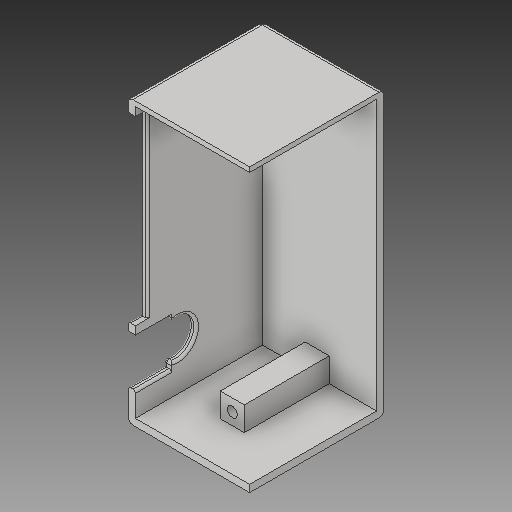
# Autodesk Inventor part: PowerS_cap
Saved by Autodesk Inventor 2019.3 (Build 233278000, 278)
## iProperties
Created: 2020-08-31
Part Number: PowerS_cap
Material: Generisch
Document SubType Name: Modeling
Designer: Nicolas Frick
Density: 1 g/cm^3
Appearance: Vorgabe
Author: Nicolas Frick
Autodesk Inventor part; units mm, degrees
ref_plane "YZ Plane" through (0, 0, 0) normal (1, 0, 0) x (0, 1, 0)
ref_plane "XZ Plane" through (0, 0, 0) normal (0, 1, 0) x (-1, 0, 0)
sketch "Skizze1" plane through (0, 0, 0) normal (0, 0, 1) x (1, 0, 0)
  line L0 (105.8135, 54.6424) -> (-70.1865, 54.6424) construction
  line L1 (-70.1865, 54.6424) -> (-70.1865, -55.3576) construction
  line L2 (-70.1865, -55.3576) -> (-86.1865, -55.3576) construction
  line L3 (-86.1865, -55.3576) -> (-86.1865, -56.6576) construction
  line L4 (112.8344, -56.6576) -> (-86.1865, -56.6576) construction
  line L5 (112.8344, -55.3576) -> (112.8344, -56.6576) construction
  line L6 (112.8344, -55.3576) -> (105.8135, -55.3576) construction
  line L7 (105.8135, -55.3576) -> (105.8135, 54.6424) construction
  line L8 (-104.5712, -45.4245) -> (-104.5712, -55.4245) construction
  line L9 (112.8135, -55.4245) -> (-104.5712, -55.4245) construction
  line L10 (112.8135, 46.962) -> (112.8135, -55.4245) construction
  line L11 (110.3928, 46.962) -> (112.8135, 46.962) construction
  arc A0 (110.3928, 50.262) -> (110.3928, 46.962) centre (110.3928, 48.612) ccw construction
  line L12 (112.8135, 50.262) -> (110.3928, 50.262) construction
  line L13 (112.8135, 54.6424) -> (112.8135, 50.262) construction
  line L14 (-86.7728, 54.6424) -> (112.8135, 54.6424) construction
  line L15 (-86.7728, 54.6424) -> (-86.7728, 44.6424) construction
  line L16 (-86.7728, 44.6424) -> (-96.7728, 44.6424) construction
  line L17 (-96.7728, 44.6424) -> (-96.7728, 54.6424) construction
  line L18 (-112.5712, 54.6424) -> (-96.7728, 54.6424) construction
  arc A1 (-112.5712, 54.6424) -> (-114.5712, 52.6424) centre (-112.5712, 52.6424) ccw construction
  line L19 (-114.5712, 44.6424) -> (-114.5712, 52.6424) construction
  line L20 (-114.5712, 44.6424) -> (-104.5712, 44.6424) construction
  line L21 (-104.5712, 44.6424) -> (-104.5712, 24.6424) construction
  line L22 (-104.5712, 24.6424) -> (-114.5712, 24.6424) construction
  line L23 (-114.5712, -45.4245) -> (-114.5712, 24.6424) construction
  line L24 (-114.5712, -45.4245) -> (-104.5712, -45.4245) construction
  circle A2 centre (-81.2226, -51.7118) radius 2 construction
  circle A3 centre (-109.5712, -50.4245) radius 1.75 construction
  arc A4 (-114.5712, -53.4245) -> (-112.5712, -55.4245) centre (-112.5712, -53.4245) ccw construction
  line L25 (-112.5712, -55.4245) -> (-104.5712, -55.4245) construction
  line L26 (-104.5712, -55.4245) -> (-104.5712, -45.4245) construction
  line L27 (-104.5712, -45.4245) -> (-114.5712, -45.4245) construction
  line L28 (-114.5712, -45.4245) -> (-114.5712, -53.4245) construction
  circle A5 centre (-91.7728, 49.6424) radius 1.75 construction
  line L29 (-86.7728, 54.6424) -> (-96.7728, 54.6424) construction
  line L30 (-96.7728, 54.6424) -> (-96.7728, 44.6424) construction
  line L31 (-96.7728, 44.6424) -> (-86.7728, 44.6424) construction
  line L32 (-86.7728, 44.6424) -> (-86.7728, 54.6424) construction
  line L33 (-114.5712, 42.6424) -> (-114.5712, 26.6424) construction
  arc A6 (-114.5712, 26.6424) -> (-112.5712, 24.6424) centre (-112.5712, 26.6424) ccw construction
  arc A7 (-112.5712, 44.6424) -> (-114.5712, 42.6424) centre (-112.5712, 42.6424) ccw construction
  line L34 (-114.5712, -56.6576) -> (-67.0712, -56.6576)
  line L35 (-67.0712, -56.6576) -> (-67.0712, 54.6424)
  line L36 (-67.0712, 54.6424) -> (-114.5712, 54.6424)
  line L37 (-114.5712, 54.6424) -> (-114.5712, -56.6576)
  point P0 (0, 0)
extrude "Extrusion1" add sketch "Skizze1" along normal blind 3
sketch "Skizze2" plane through (0, 0, 0) normal (0, 0, -1) x (-1, 0, 0)
  line L0 (104.5712, 43.4093) -> (114.5712, 43.4093) projected
  line L1 (104.5712, 53.4093) -> (104.5712, 43.4093) projected
  line L2 (112.5712, 53.4093) -> (104.5712, 53.4093) projected
  circle A0 centre (109.5712, 48.4093) radius 1.75 projected
  line L3 (114.5712, 54.6424) -> (114.5712, -56.6576) projected
  circle A1 centre (91.7728, -51.6576) radius 1.75 projected
  line L4 (86.7728, -46.6576) -> (86.7728, -56.6576) projected
  line L5 (114.5712, -56.6576) -> (67.0712, -56.6576) projected
  line L6 (96.7728, -46.6576) -> (86.7728, -46.6576) projected
  line L7 (96.7728, -56.6576) -> (96.7728, -46.6576) projected
  line L8 (114.5712, 54.6424) -> (114.5712, -56.6576) projected
  line L9 (104.5712, 43.4093) -> (114.5712, 43.4093)
  line L10 (114.5712, 43.4093) -> (114.5712, 53.4093)
  line L11 (114.5712, 53.4093) -> (104.5712, 53.4093)
  line L12 (104.5712, 53.4093) -> (104.5712, 43.4093)
  line L13 (86.7728, -56.6576) -> (96.7728, -56.6576)
  line L14 (96.7728, -56.6576) -> (96.7728, -46.6576)
  line L15 (96.7728, -46.6576) -> (86.7728, -46.6576)
  line L16 (86.7728, -46.6576) -> (86.7728, -56.6576)
  circle A2 centre (91.7728, -51.6576) radius 2.1
  circle A3 centre (109.5712, 48.4093) radius 2.1
  point P0 (0, 0)
  dimension "d3" = 4.2
  dimension "d4" = 4.2
  constraints: 16 end point, 4 parallel, 2 centre point, 2 coincident, 2 horizontal, 2 perpendicular, 1 point on line
  measures "d3" diameter of A2
  measures "d4" diameter of A3
ref_plane "Arbeitsebene1" through (-114.5712, 43.4093, 38.3) normal (0, 0, -1) x (0, 1, 0)
extrude "Extrusion2" add sketch "Skizze2" against normal up to surface (38.3 mm away) contours L1 L2 L11 L3 L0 | L5 L4 L6 L7
sketch "Skizze3" plane through (0, 0, 0) normal (0, 0, -1) x (-1, 0, 0)
  circle A0 centre (91.7728, -51.6576) radius 2.1 projected
  circle A1 centre (109.5712, 48.4093) radius 2.1 projected
  point P0 (0, 0)
hole "Bohrung1" at (-109.5712, 48.4093, 0) at (-91.7728, -51.6576, 0) direction (0, 0, 1) diameter 4.2 depth 38.3 counterbore diameter 8 counterbore depth 25
fillet "Rundung1" radius 1 2 edges at (-91.7728, -55.6576, 0) (-109.5712, 44.4093, 0)
sketch "Skizze4" plane through (-114.5712, 54.6424, 0) normal (-1, 0, 0) x (0, 0, 1)
  line L0 (3, 0) -> (3, -1.2331) construction
  line L1 (0, 0) -> (3, 0) construction
  line L2 (0, 0) -> (0, -6.2331) construction
  line L3 (0, -6.2331) -> (0, -111.3) construction
  line L4 (0, -111.3) -> (3, -111.3) construction
  line L5 (3, -11.2331) -> (3, -111.3) construction
  line L6 (3, -11.2331) -> (38.3, -11.2331) construction
  line L7 (38.3, -1.2331) -> (38.3, -11.2331) construction
  line L8 (3, -1.2331) -> (38.3, -1.2331) construction
  line L9 (25, -102.3) -> (1, -102.3) construction
  line L10 (3, -111.3) -> (38.3, -111.3) construction
  line L11 (55.8, -3.2331) -> (55.8, -109.3) construction
  line L12 (0, -111.3) -> (55.8, -111.3)
  line L13 (55.8, -111.3) -> (55.8, 0)
  line L14 (55.8, 0) -> (0, 0)
  line L15 (0, 0) -> (0, -111.3)
  point P0 (0, -54.6424)
  constraints: 8 end point, 2 parallel, 1 horizontal, 1 perpendicular
extrude "Extrusion4" add sketch "Skizze4" along normal blind 3
sketch "Skizze5" plane through (-67.0712, 54.6424, 3) normal (0, 1, 0) x (1, 0, 0)
  line L0 (0, 3) -> (-50.5, 3) construction
  line L1 (-50.5, -52.8) -> (-50.5, 3) construction
  line L2 (179.8847, -52.8) -> (-45.5, -52.8) construction
  line L3 (-50.5, 3) -> (0, 3)
  line L4 (0, 3) -> (0, -52.8)
  line L5 (0, -52.8) -> (-50.5, -52.8)
  line L6 (-50.5, -52.8) -> (-50.5, 3)
  point P0 (67.0712, 3)
  constraints: 8 end point, 2 parallel, 1 horizontal, 1 perpendicular, 1 point on line
extrude "Extrusion5" add sketch "Skizze5" along normal blind 3
fillet "Rundung2" radius 2 1 edges at (-117.5712, 57.6424, 27.9)
sketch "Skizze6" plane through (-67.0712, -56.6576, 0) normal (0, -1, 0) x (1, 0, 0)
  line L0 (-47.5, 3) -> (-29.7016, 3) construction
  line L1 (-47.5, 3) -> (-47.5, 55.8) construction
  line L2 (-47.5, 55.8) -> (-50.5, 55.8) construction
  line L3 (-50.5, 0) -> (-50.5, 55.8) construction
  line L4 (-50.5, 0) -> (-24.7016, 0) construction
  line L5 (-24.7016, 0) -> (0, 0) construction
  line L6 (0, 0) -> (0, 3) construction
  line L7 (-19.7016, 3) -> (0, 3) construction
  line L8 (-19.7016, 3) -> (-19.7016, 38.3) construction
  line L9 (-29.7016, 38.3) -> (-19.7016, 38.3) construction
  line L10 (-29.7016, 3) -> (-29.7016, 38.3) construction
  line L11 (0, 3) -> (0, 55.8) construction
  line L12 (-45.5, 55.8) -> (179.8847, 55.8) construction
  line L13 (-50.5, 55.8) -> (-48.5, 55.8) projected
  line L14 (0, 0) -> (-50.5, 0)
  line L15 (-50.5, 0) -> (-50.5, 55.8)
  line L16 (-50.5, 55.8) -> (0, 55.8)
  line L17 (0, 55.8) -> (0, 0)
  point P0 (67.0712, 0)
  constraints: 8 end point, 2 parallel, 1 horizontal, 1 perpendicular
extrude "Extrusion6" add sketch "Skizze6" along normal blind 3
fillet "Rundung3" radius 2 3 edges at (-92.3212, -59.6576, 0) (-117.5712, -59.6576, 27.9) (-91.3212, 57.6424, 0)
sketch "Skizze7" plane through (0, 0, 3) normal (0, 0, 1) x (1, 0, 0)
  arc A0 (-117.5712, -57.6576) -> (-115.5712, -59.6576) centre (-115.5712, -57.6576) ccw construction
  line L0 (-67.0712, -59.6576) -> (-115.5712, -59.6576) construction
  line L1 (-67.0712, -56.6576) -> (-67.0712, -59.6576) construction
  line L2 (-67.0712, -56.6576) -> (-114.5712, -56.6576) construction
  line L3 (-114.5712, -56.6576) -> (-114.5712, 54.6424) construction
  line L4 (-67.0712, 54.6424) -> (-114.5712, 54.6424) construction
  line L5 (-67.0712, 54.6424) -> (-67.0712, 57.6424) construction
  line L6 (-115.5712, 57.6424) -> (-67.0712, 57.6424) construction
  arc A1 (-115.5712, 57.6424) -> (-117.5712, 55.6424) centre (-115.5712, 55.6424) ccw construction
  line L7 (-117.5712, 55.6424) -> (-117.5712, -57.6576) construction
  line L8 (112.8135, 53.4093) -> (-112.5712, 53.4093) construction
  line L9 (-67.0712, 54.6424) -> (-114.5712, 54.6424) construction
  line L10 (-67.0712, 55.6424) -> (-115.5712, 55.6424) projected
  line L11 (-67.0712, 54.6424) -> (-114.5712, 54.6424)
  line L12 (-114.5712, 54.6424) -> (-114.5712, 55.6424)
  line L13 (-114.5712, 55.6424) -> (-67.0712, 55.6424)
  line L14 (-67.0712, 55.6424) -> (-67.0712, 54.6424)
  point P0 (0, 0)
  constraints: 8 end point, 2 parallel, 1 horizontal, 1 perpendicular, 1 point on line
extrude "Extrusion7" cut sketch "Skizze7" along normal up to surface (52.8 mm away)
sketch "Skizze9" plane through (-117.5712, 54.6424, 0) normal (-1, 0, 0) x (0, 0, 1)
  line L0 (2, -112.3) -> (2, 1) construction
  line L1 (55.8, -112.3) -> (2, -112.3) construction
  line L2 (55.8, 1) -> (55.8, -112.3) construction
  line L3 (2, 1) -> (55.8, 1) construction
  line L4 (52.8, -101.3) -> (38.3, -101.3) construction
  line L5 (52.8, -81.3) -> (38.3, -81.3) construction
  line L6 (36.3, -99.3) -> (36.3, -83.3) construction
  line L7 (55.8, -111.3) -> (55.8, 1) construction
  line L8 (55.8, -101.3) -> (50.8, -101.3)
  line L9 (50.8, -77.9589) -> (50.8, -2.6275)
  line L10 (50.8, -2.6275) -> (55.8, -2.6275)
  line L11 (50.8, -101.3) -> (40.8, -101.3)
  line L12 (40.8, -101.3) -> (40.8, -81.3)
  line L13 (40.8, -81.3) -> (50.8, -81.3)
  line L14 (50.8, -81.3) -> (55.8, -81.3)
  line L15 (55.8, -77.9589) -> (50.8, -77.9589)
  line L16 (55.8, -2.6275) -> (55.8, -77.9589)
  line L17 (55.8, -81.3) -> (55.8, -101.3)
  point P0 (0, -54.6424)
  dimension "d31" = 5
  constraints: 20 end point, 5 parallel, 3 horizontal, 2 perpendicular, 2 point on line
  measures "d31" distance of L9.end L10.end
extrude "Extrusion9" cut sketch "Skizze9" against normal blind 3
fillet "Rundung4" radius 1 8 edges at (-117.5712, -46.6576, 48.3) (-117.5712, -36.6576, 40.8) (-114.5712, -46.6576, 48.3) (-117.5712, -23.3164, 53.3) (-117.5712, -26.6576, 48.3) (-117.5712, 14.3492, 50.8) (-114.5712, 14.3492, 50.8) (-117.5712, 52.0149, 53.3)
sketch "Skizze10" plane through (-117.5712, 54.6424, 0) normal (-1, 0, 0) x (0, 0, 1)
  line L0 (38.3, -3.2331) -> (55.8, -3.2331) construction
  line L1 (38.3, -11.2331) -> (38.3, -3.2331) construction
  line L2 (52.8, -11.2331) -> (38.3, -11.2331) construction
  line L3 (52.8, -11.2331) -> (52.8, -81.3) construction
  line L4 (52.8, -81.3) -> (38.3, -81.3) construction
  line L5 (38.3, -87.2689) -> (38.3, -81.3) construction
  arc A0 (38.3, -87.2689) -> (39.4111, -89.0605) centre (40.3, -87.2689) ccw construction
  arc A1 (40.7863, -91.0383) -> (39.4111, -89.0605) centre (38.3, -91.3) ccw construction
  line L6 (40.4663, -91.0383) -> (40.7863, -91.0383) construction
  line L7 (40.4663, -91.0383) -> (40.4663, -91.5741) construction
  line L8 (40.4663, -91.5741) -> (40.7849, -91.5741) construction
  arc A2 (39.4111, -93.5395) -> (40.7849, -91.5741) centre (38.3, -91.3) ccw construction
  arc A3 (39.4111, -93.5395) -> (38.3, -95.3311) centre (40.3, -95.3311) ccw construction
  line L9 (38.3, -101.3) -> (38.3, -95.3311) construction
  line L10 (52.8, -101.3) -> (38.3, -101.3) construction
  line L11 (52.8, -101.3) -> (52.8, -109.3) construction
  line L12 (55.8, -109.3) -> (52.8, -109.3) construction
  line L13 (55.8, -3.2331) -> (55.8, -109.3) construction
  arc A4 (40.8, -83.9404) -> (40.8, -98.6596) centre (38.3, -91.3) ccw
  line L14 (40.8, -101.3) -> (40.8, -81.3) projected
  line L15 (40.8, -98.6596) -> (40.8, -83.9404)
  point P0 (0, -54.6424)
  constraints: 2 end point, 2 point on circle, 2 point on line, 1 centre point, 1 coincident
extrude "Extrusion10" cut sketch "Skizze10" against normal blind 3
fillet "Rundung5" radius 1 6 edges at (-114.5712, -36.6576, 30.5274) (-117.2456, -29.2142, 40.5383) (-117.2456, -44.1009, 40.5383) (-115.5712, -29.298, 40.8) (-115.5712, -44.0172, 40.8) (-117.5712, -36.6576, 30.5274)
